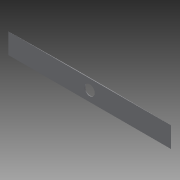
# Autodesk Inventor part: lama
Saved by Autodesk Inventor 2014 SP2 (Build 180246200, 246)
## iProperties
Created: 2019-04-05
Part Number: lama
Material: Generic
Document SubType Name: Modeling
Designer: GauchoHP
Density: 1 g/cm^3
Appearance: Default
Author: GauchoHP
Autodesk Inventor part; units mm, degrees
ref_plane "YZ Plane" through (0, 0, 0) normal (1, 0, 0) x (0, 1, 0)
ref_plane "XZ Plane" through (0, 0, 0) normal (0, 1, 0) x (-1, 0, 0)
ref_plane "XY Plane" through (0, 0, 0) normal (0, 0, 1) x (1, 0, 0)
sketch "Sketch1" plane through (0, 0, 0) normal (0, 1, 0) x (-1, 0, 0)
  line L0 (-143.1635, -20.2145) -> (110.8365, -20.2145)
  line L1 (110.8365, -20.2145) -> (110.8365, -52.2145)
  line L2 (110.8365, -52.2145) -> (-143.1635, -52.2145)
  line L3 (-143.1635, -52.2145) -> (-143.1635, -20.2145)
  circle A0 centre (-16.1635, -36.2145) radius 8
  point P0 (0, 0)
  dimension "d0" = 254
  dimension "d1" = 32
  dimension "d10" = 16
  dimension "d11" = 127
  dimension "d12" = 16
  constraints: 8 end point, 2 parallel, 1 centre point, 1 horizontal, 1 perpendicular
  measures "d0" distance of L1.end L2.end
  measures "d1" distance of L2.end L0.start
  measures "d10" diameter of A0
  measures "d11" distance from line of L3 A0.centre
  measures "d12" distance from line of L0 A0.centre
extrude "Extrusion1" add sketch "Sketch1" along normal blind 1
chamfer "Chamfer1" distance 100 distance2 1 1 edges at (143.1635, 1, -36.2145) measured on face at (103.4969, 1, -36.2145)
chamfer "Chamfer2" distance 100 distance2 1 1 edges at (-110.8365, 1, -36.2145) measured on face at (-71.1698, 1, -36.2145)
body "Solid1"
